Autodesk Inventor part; units mm, degrees
(part 2 of 2)
  spline S256 degree 2 poles (-40.0251, 66.1089) (-39.9054, 66.7538) (-39.4601, 67.612) (-39.0491, 67.8632) knots 0 0 0 1 2 2 2
  spline S257 degree 2 poles (-39.0491, 67.8632) (-38.733, 68.0564) (-38.0974, 68.177) (-37.7725, 68.0716) knots 0 0 0 1 2 2 2
  spline S258 degree 2 poles (-37.7725, 68.0716) (-37.4423, 67.9694) (-36.8206, 67.4375) (-36.5147, 66.937) knots 0 0 0 1 2 2 2
  line L277 (-36.5147, 66.937) -> (-34.5506, 63.7228)
  line L278 (-34.5506, 63.7228) -> (-35.3726, 63.2205)
  spline S259 degree 2 poles (-31.0338, 65.2582) (-32.2683, 64.6623) (-34.2937, 65.3919) (-34.9111, 66.6709) knots 0 0 0 1 2 2 2
  spline S260 degree 2 poles (-34.9111, 66.6709) (-35.5178, 67.9277) (-34.9193, 70.0543) (-33.8572, 70.567) knots 0 0 0 1 2 2 2
  spline S261 degree 2 poles (-33.8572, 70.567) (-33.379, 70.7979) (-32.5051, 70.8769) (-32.0903, 70.7137) knots 0 0 0 1 2 2 2
  spline S262 degree 2 poles (-32.0903, 70.7137) (-31.67, 70.5532) (-30.9645, 69.8447) (-30.6666, 69.2274) knots 0 0 0 1 2 2 2
  line L279 (-30.6666, 69.2274) -> (-30.4384, 68.7547)
  line L280 (-30.4384, 68.7547) -> (-34.0029, 67.0339)
  spline S263 degree 2 poles (-34.0029, 67.0339) (-33.5707, 66.1386) (-32.2108, 65.6226) (-31.41, 66.0092) knots 0 0 0 1 2 2 2
  spline S264 degree 2 poles (-31.41, 66.0092) (-31.1264, 66.1461) (-30.6376, 66.5397) (-30.4635, 66.7472) knots 0 0 0 1 2 2 2
  spline S265 degree 2 poles (-30.4635, 66.7472) (-30.2836, 66.9712) (-30.0551, 67.3215) (-29.9924, 67.4615) knots 0 0 0 1 2 2 2
  line L281 (-29.9924, 67.4615) -> (-29.9423, 67.4857)
  line L282 (-29.9423, 67.4857) -> (-29.4859, 66.5403)
  spline S266 degree 2 poles (-29.4859, 66.5403) (-29.6065, 66.4067) (-29.9766, 66.0086) (-30.1304, 65.8726) knots 0 0 0 1 2 2 2
  spline S267 degree 2 poles (-30.1304, 65.8726) (-30.3458, 65.6795) (-30.7224, 65.4086) (-31.0338, 65.2582) knots 0 0 0 1 2 2 2
  spline S268 degree 2 poles (-31.6031, 69.0084) (-31.7834, 69.3534) (-32.1749, 69.7952) (-32.3972, 69.9005) knots 0 0 0 1 2 2 2
  spline S269 degree 2 poles (-32.3972, 69.9005) (-32.6413, 70.0226) (-33.2133, 70.0002) (-33.5636, 69.8311) knots 0 0 0 1 2 2 2
  spline S270 degree 2 poles (-33.5636, 69.8311) (-33.9084, 69.6646) (-34.2929, 69.2253) (-34.3964, 68.9285) knots 0 0 0 1 2 2 2
  spline S271 degree 2 poles (-34.3964, 68.9285) (-34.4917, 68.6288) (-34.453, 68.0372) (-34.3224, 67.6957) knots 0 0 0 1 2 2 2
  line L283 (-34.3224, 67.6957) -> (-31.6031, 69.0084)
  spline S272 degree 2 poles (-26.6867, 67.1752) (-27.4128, 66.8789) (-28.5687, 67.3742) (-28.935, 68.2718) knots 0 0 0 1 2 2 2
  line L284 (-28.935, 68.2718) -> (-30.132, 71.2048)
  line L285 (-30.132, 71.2048) -> (-30.7323, 70.9598)
  line L286 (-30.7323, 70.9598) -> (-31.0332, 71.6973)
  line L287 (-31.0332, 71.6973) -> (-30.4329, 71.9423)
  line L288 (-30.4329, 71.9423) -> (-31.0536, 73.4631)
  line L289 (-31.0536, 73.4631) -> (-30.1617, 73.8271)
  line L290 (-30.1617, 73.8271) -> (-29.541, 72.3063)
  line L291 (-29.541, 72.3063) -> (-27.9002, 72.9759)
  line L292 (-27.9002, 72.9759) -> (-27.5992, 72.2384)
  line L293 (-27.5992, 72.2384) -> (-29.2401, 71.5688)
  line L294 (-29.2401, 71.5688) -> (-28.2111, 69.0475)
  spline S273 degree 2 poles (-28.2111, 69.0475) (-28.0478, 68.6472) (-27.8396, 68.2187) (-27.6654, 68.0697) knots 0 0 0 1 2 2 2
  spline S274 degree 2 poles (-27.6654, 68.0697) (-27.5177, 67.9365) (-27.0898, 67.9177) (-26.7811, 68.0437) knots 0 0 0 1 2 2 2
  spline S275 degree 2 poles (-26.7811, 68.0437) (-26.5638, 68.1324) (-26.2116, 68.4295) (-26.1364, 68.5069) knots 0 0 0 1 2 2 2
  line L295 (-26.1364, 68.5069) -> (-26.085, 68.5279)
  line L296 (-26.085, 68.5279) -> (-25.7583, 67.7275)
  spline S276 degree 2 poles (-25.7583, 67.7275) (-25.9819, 67.5562) (-26.4638, 67.2662) (-26.6867, 67.1752) knots 0 0 0 1 2 2 2
  spline S277 degree 2 poles (-22.6844, 68.6087) (-23.9834, 68.1707) (-25.9024, 69.1464) (-26.3561, 70.4922) knots 0 0 0 1 2 2 2
  spline S278 degree 2 poles (-26.3561, 70.4922) (-26.802, 71.8146) (-25.9439, 73.8504) (-24.8262, 74.2272) knots 0 0 0 1 2 2 2
  spline S279 degree 2 poles (-24.8262, 74.2272) (-24.323, 74.3968) (-23.4461, 74.3666) (-23.0549, 74.1532) knots 0 0 0 1 2 2 2
  spline S280 degree 2 poles (-23.0549, 74.1532) (-22.6577, 73.9417) (-22.0458, 73.151) (-21.8268, 72.5015) knots 0 0 0 1 2 2 2
  line L297 (-21.8268, 72.5015) -> (-21.6591, 72.0041)
  line L298 (-21.6591, 72.0041) -> (-25.4099, 70.7395)
  spline S281 degree 2 poles (-25.4099, 70.7395) (-25.0923, 69.7975) (-23.807, 69.1165) (-22.9644, 69.4005) knots 0 0 0 1 2 2 2
  spline S282 degree 2 poles (-22.9644, 69.4005) (-22.666, 69.5011) (-22.132, 69.831) (-21.9335, 70.0153) knots 0 0 0 1 2 2 2
  spline S283 degree 2 poles (-21.9335, 70.0153) (-21.7272, 70.2152) (-21.4569, 70.5344) (-21.3772, 70.6655) knots 0 0 0 1 2 2 2
  line L299 (-21.3772, 70.6655) -> (-21.3246, 70.6832)
  line L300 (-21.3246, 70.6832) -> (-20.9892, 69.6885)
  spline S284 degree 2 poles (-20.9892, 69.6885) (-21.1255, 69.5709) (-21.5422, 69.2218) (-21.7117, 69.1061) knots 0 0 0 1 2 2 2
  spline S285 degree 2 poles (-21.7117, 69.1061) (-21.9494, 68.9412) (-22.3567, 68.7192) (-22.6844, 68.6087) knots 0 0 0 1 2 2 2
  spline S286 degree 2 poles (-22.7833, 72.4006) (-22.9193, 72.7652) (-23.2529, 73.2523) (-23.4603, 73.3844) knots 0 0 0 1 2 2 2
  spline S287 degree 2 poles (-23.4603, 73.3844) (-23.6874, 73.5359) (-24.2577, 73.5847) (-24.6264, 73.4604) knots 0 0 0 1 2 2 2
  spline S288 degree 2 poles (-24.6264, 73.4604) (-24.9892, 73.3381) (-25.4253, 72.95) (-25.5649, 72.6683) knots 0 0 0 1 2 2 2
  spline S289 degree 2 poles (-25.5649, 72.6683) (-25.6967, 72.3828) (-25.7318, 71.791) (-25.6446, 71.4359) knots 0 0 0 1 2 2 2
  line L301 (-25.6446, 71.4359) -> (-22.7833, 72.4006)
  line L302 (-18.1122, 74.9412) -> (-18.1599, 74.9284)
  spline S290 degree 2 poles (-18.1599, 74.9284) (-18.2752, 74.9296) (-18.5111, 74.8793) (-18.6722, 74.8363) knots 0 0 0 1 2 2 2
  spline S291 degree 2 poles (-18.6722, 74.8363) (-19.048, 74.7359) (-19.7002, 74.2102) (-19.9482, 73.7988) knots 0 0 0 1 2 2 2
  line L303 (-19.9482, 73.7988) -> (-18.9013, 69.8792)
  line L304 (-18.9013, 69.8792) -> (-19.8319, 69.6306)
  line L305 (-19.8319, 69.6306) -> (-21.3075, 75.1551)
  line L306 (-21.3075, 75.1551) -> (-20.3768, 75.4036)
  line L307 (-20.3768, 75.4036) -> (-20.1569, 74.5804)
  spline S292 degree 2 poles (-20.1569, 74.5804) (-19.7709, 75.1692) (-19.1121, 75.7415) (-18.7541, 75.8371) knots 0 0 0 1 2 2 2
  spline S293 degree 2 poles (-18.7541, 75.8371) (-18.6109, 75.8753) (-18.4646, 75.9016) (-18.3703, 75.9076) knots 0 0 0 1 2 2 2
  line L308 (-18.3703, 75.9076) -> (-18.1122, 74.9412)
  spline S294 degree 2 poles (-8.9302, 77.2452) (-8.8565, 76.7568) (-9.0718, 75.825) (-9.3372, 75.4727) knots 0 0 0 1 2 2 2
  spline S295 degree 2 poles (-9.3372, 75.4727) (-9.6699, 75.029) (-10.6663, 74.4727) (-11.4723, 74.3511) knots 0 0 0 1 2 2 2
  line L309 (-11.4723, 74.3511) -> (-12.321, 74.2229)
  line L310 (-12.321, 74.2229) -> (-11.897, 71.4142)
  line L311 (-11.897, 71.4142) -> (-12.8984, 71.2631)
  line L312 (-12.8984, 71.2631) -> (-14.0357, 78.7978)
  line L313 (-14.0357, 78.7978) -> (-12.1428, 79.0835)
  spline S296 degree 2 poles (-12.1428, 79.0835) (-11.4712, 79.1848) (-10.4977, 79.107) (-10.0997, 78.911) knots 0 0 0 1 2 2 2
  spline S297 degree 2 poles (-10.0997, 78.911) (-9.6351, 78.6876) (-9.0252, 77.8741) (-8.9302, 77.2452) knots 0 0 0 1 2 2 2
  spline S298 degree 2 poles (-9.9697, 77.0571) (-10.0287, 77.4479) (-10.384, 77.9813) (-10.6864, 78.123) knots 0 0 0 1 2 2 2
  spline S299 degree 2 poles (-10.6864, 78.123) (-10.9485, 78.2458) (-11.6029, 78.2782) (-12.073, 78.2072) knots 0 0 0 1 2 2 2
  line L314 (-12.073, 78.2072) -> (-12.9034, 78.0819)
  line L315 (-12.9034, 78.0819) -> (-12.45, 75.0778)
  line L316 (-12.45, 75.0778) -> (-11.7661, 75.181)
  spline S300 degree 2 poles (-11.7661, 75.181) (-11.1556, 75.2732) (-10.434, 75.5819) (-10.2285, 75.8752) knots 0 0 0 1 2 2 2
  spline S301 degree 2 poles (-10.2285, 75.8752) (-10.0367, 76.1352) (-9.9154, 76.6969) (-9.9697, 77.0571) knots 0 0 0 1 2 2 2
  line L317 (-2.1666, 80.0418) -> (-4.2817, 72.265)
  line L318 (-4.2817, 72.265) -> (-5.3723, 72.1928)
  line L319 (-5.3723, 72.1928) -> (-8.4945, 79.6227)
  line L320 (-8.4945, 79.6227) -> (-7.4101, 79.6945)
  line L321 (-7.4101, 79.6945) -> (-4.8846, 73.5185)
  line L322 (-4.8846, 73.5185) -> (-3.1956, 79.9736)
  line L323 (-3.1956, 79.9736) -> (-2.1666, 80.0418)
  spline S302 degree 2 poles (3.743, 76.1471) (3.7079, 74.0973) (2.4834, 72.1975) (1.2424, 72.2188) knots 0 0 0 1 2 2 2
  spline S303 degree 2 poles (1.2424, 72.2188) (-0.0171, 72.2403) (-1.1629, 74.2177) (-1.1285, 76.2243) knots 0 0 0 1 2 2 2
  spline S304 degree 2 poles (-1.1285, 76.2243) (-1.0932, 78.2865) (0.1311, 80.1739) (1.3782, 80.1525) knots 0 0 0 1 2 2 2
  spline S305 degree 2 poles (1.3782, 80.1525) (2.6316, 80.1311) (3.777, 78.1352) (3.743, 76.1471) knots 0 0 0 1 2 2 2
  spline S306 degree 2 poles (2.3943, 73.848) (2.549, 74.2221) (2.6923, 75.3807) (2.7057, 76.1648) knots 0 0 0 1 2 2 2
  spline S307 degree 2 poles (2.7057, 76.1648) (2.7192, 76.949) (2.6154, 78.1056) (2.4677, 78.4973) knots 0 0 0 1 2 2 2
  spline S308 degree 2 poles (2.4677, 78.4973) (2.3201, 78.8889) (1.7898, 79.2994) (1.3638, 79.3067) knots 0 0 0 1 2 2 2
  spline S309 degree 2 poles (1.3638, 79.3067) (0.9377, 79.314) (0.3814, 78.9221) (0.214, 78.5235) knots 0 0 0 1 2 2 2
  spline S310 degree 2 poles (0.214, 78.5235) (0.053, 78.1372) (-0.0785, 76.9536) (-0.0912, 76.2065) knots 0 0 0 1 2 2 2
  spline S311 degree 2 poles (-0.0912, 76.2065) (-0.105, 75.4039) (-0.0246, 74.3279) (0.1287, 73.9053) knots 0 0 0 1 2 2 2
  spline S312 degree 2 poles (0.1287, 73.9053) (0.2702, 73.5077) (0.8124, 73.0722) (1.2569, 73.0646) knots 0 0 0 1 2 2 2
  spline S313 degree 2 poles (1.2569, 73.0646) (1.6767, 73.0574) (2.2331, 73.4493) (2.3943, 73.848) knots 0 0 0 1 2 2 2
  line L324 (9.7823, 74.413) -> (8.8788, 74.5001)
  line L325 (8.8788, 74.5001) -> (8.6276, 71.8939)
  line L326 (8.6276, 71.8939) -> (7.6503, 71.9881)
  line L327 (7.6503, 71.9881) -> (7.9015, 74.5943)
  line L328 (7.9015, 74.5943) -> (4.5516, 74.9171)
  line L329 (4.5516, 74.9171) -> (4.6547, 75.9866)
  line L330 (4.6547, 75.9866) -> (8.4243, 79.5688)
  line L331 (8.4243, 79.5688) -> (9.3585, 79.4788)
  line L332 (9.3585, 79.4788) -> (8.9576, 75.3176)
  line L333 (8.9576, 75.3176) -> (9.8611, 75.2305)
  line L334 (9.8611, 75.2305) -> (9.7823, 74.413)
  line L335 (7.9803, 75.4118) -> (8.2657, 78.3744)
  line L336 (8.2657, 78.3744) -> (5.4294, 75.6576)
  line L337 (5.4294, 75.6576) -> (7.9803, 75.4118)
  dimension "d18" = 152.4
  constraints: 1 centre point, 1 coincident, 1 other
  measures "d18" diameter of A0
extrude "ExtrusionForText" cut sketch "Sketch5" against normal blind 1.27
sketch "Sketch13" plane through (0, -9.525, 0) normal (0, -1, 0) x (1, 0, 0)
  point P0 (0, 0)
  point P1 (44.45, 0)
  point P2 (22.225, 38.4948)
  point P3 (-22.225, 38.4948)
  point P4 (-44.45, 0)
  point P5 (-22.225, -38.4948)
  point P6 (22.225, -38.4948)
  dimension "d65" = 44.45
  dimension "d68" = 360
  constraints: 7 other
  measures "d65" distance of point (44.45, 0) point (0, 0)
hole "Hole6" at (44.45, -9.525, 0) at (22.225, -9.525, 38.4948) at (-22.225, -9.525, 38.4948) at (-44.45, -9.525, 0) at (-22.225, -9.525, -38.4948) at (22.225, -9.525, -38.4948) direction (0, 1, 0) diameter 6.3246 end through all counterbore diameter 7.0891 counterbore depth 6.1239
fillet "Fillet2" radius 1.27 1 edges at (10.795, -44.525, 0)
sketch "Sketch16" plane through (0, 0, 0) normal (0, 1, 0) x (1, 0, 0)
  point P0 (0, 0)
  point P1 (0, 0)
  constraints: 1 coincident
hole "Hole7" at (0, 0, 0) direction (0, -1, 0) diameter 11.9888 end through all clearance for "Flat Head Machine Screw" size "M10" standard "Ansi Metric M Profile"
sketch "Sketch18" plane through (0, 0, 0) normal (0, 1, 0) x (1, 0, 0)
  line L0 (9.9616, 0) -> (4.9808, -8.627)
  line L1 (4.9808, -8.627) -> (-4.9808, -8.627)
  line L2 (-4.9808, -8.627) -> (-9.9616, 0)
  line L3 (-9.9616, 0) -> (-4.9808, 8.627)
  line L4 (-4.9808, 8.627) -> (4.9808, 8.627)
  line L5 (4.9808, 8.627) -> (9.9616, 0)
  point P0 (0, 0)
  point P1 (0, 0)
  dimension "d104" = 17.254
  constraints: 12 end point, 1 coincident, 1 horizontal, 13 other
  measures "d104" distance between parallel lines of L1 L4
extrude "Extrusion8" cut sketch "Sketch18" against normal blind 33.4
equation "\"d18\" = textDiameter"
equation "\"d0\" = topRadius"
equation "\"d3\" = topThickness"
equation "\"d4\" = depthIntoTripod"
equation "\"depthIntoTripod\" = 35"
equation "\"insertionPointDiameter\" = 25.4"
equation "\"topDiameter\" = 203.2"
equation "\"topRadius\" = 0.5 * topDiameter"
equation "\"topThickness\" = 9.525"
equation "\"hexBoltClearance\" = 17.635"
equation "\"totalPartHeight\" = depthIntoTripod + topThickness"
equation "\"hexBoltDepth\" = totalPartHeight - hexBoltSupport"
equation "\"hexBoltSupport\" = 9.525"
equation "\"holeForGearBoxHardware\" = 50.8"
equation "\"depthForGearBoxHardware\" = 6.35"
equation "\"textDiameter\" = 152.4"
body "Solid1"
